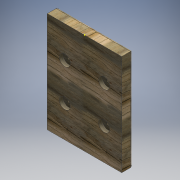
# Autodesk Inventor part: Base
Saved by Autodesk Inventor 2016 (Build 200138000, 138)
## iProperties
Created: 2016-09-10
Part Number: Base
Material: Generic
Document SubType Name: Modeling
Designer: Muhammad
Density: 1 g/cm^3
Appearance: Driftwood
Author: Muhammad
Autodesk Inventor part; units mm, degrees
ref_plane "YZ Plane" through (0, 0, 0) normal (1, 0, 0) x (0, 1, 0)
ref_plane "XZ Plane" through (0, 0, 0) normal (0, 1, 0) x (-1, 0, 0)
ref_plane "XY Plane" through (0, 0, 0) normal (0, 0, 1) x (1, 0, 0)
sketch "Sketch1" plane through (0, 0, 0) normal (0, 1, 0) x (-1, 0, 0)
  line L0 (85, 115) -> (-85, 115)
  line L1 (-85, 115) -> (-85, -115)
  line L2 (-85, -115) -> (85, -115)
  line L3 (85, -115) -> (85, 115)
  line L4 (85, 115) -> (-85, -115) construction
  line L5 (-85, 115) -> (85, -115) construction
  line L6 (-85, 115) -> (-85, 42.5) construction
  line L7 (-85, 42.5) -> (-85, -42.5) construction
  line L8 (-85, 42.5) -> (-45, 42.5) construction
  line L9 (-45, 42.5) -> (45, 42.5) construction
  line L10 (45, 42.5) -> (45, -42.5) construction
  line L11 (-85, -42.5) -> (-45, -42.5) construction
  line L12 (-45, -42.5) -> (45, -42.5) construction
  circle A0 centre (-45, 42.5) radius 3.5
  circle A1 centre (45, 42.5) radius 3.5
  circle A2 centre (45, -42.5) radius 3.5
  line L13 (-45, 42.5) -> (-45, -42.5) construction
  circle A3 centre (-45, -42.5) radius 3.5
  point P0 (0, 0)
  dimension "d3" = 85
  dimension "d7" = 7
  dimension "d8" = 7
  constraints: 28 end point, 4 centre point, 4 coincident, 4 perpendicular, 3 horizontal, 3 point on line, 2 midpoint, 2 parallel
  measures "d3" distance of L6.end L7.end
  measures "d7" diameter of A1
  measures "d8" diameter of A2
extrude "Extrusion1" add sketch "Sketch1" along normal blind 25
sketch "Sketch2" plane through (0, 0, 0) normal (0, -1, 0) x (1, 0, 0)
  circle A0 centre (-45, -42.5) radius 3.5 projected
  circle A1 centre (-45, -42.5) radius 12.5
  circle A2 centre (-45, 42.5) radius 3.5 projected
  circle A3 centre (-45, 42.5) radius 12.5
  circle A4 centre (45, 42.5) radius 3.5 projected
  circle A5 centre (45, 42.5) radius 12.5
  circle A6 centre (45, -42.5) radius 3.5 projected
  circle A7 centre (45, -42.5) radius 12.5
  point P0 (0, 0)
  constraints: 4 centre point, 4 coincident
extrude "Extrusion2" cut sketch "Sketch2" against normal blind 9
sketch "Sketch3" plane through (-85, 0, 115) normal (0, 0, 1) x (1, 0, 0)
  point P0 (85, 0)
sketch "Sketch4" plane through (0, 0, 0) normal (0, 0, 1) x (1, 0, 0)
  line L0 (-85, 0) -> (-85, 25) projected
  line L1 (-85, 7.3168) -> (-67.3168, 25)
  line L2 (-85, 25) -> (85, 25) projected
  line L3 (-85, 7.3168) -> (-59.9922, 7.3168) construction
  point P0 (0, 0)
  dimension "d15" = 45
  constraints: 4 end point, 2 point on line, 1 equal length, 1 horizontal
  measures "d15" angle of L3 L1
extrude "Extrusion3" cut sketch "Sketch4" along normal mid plane 80
fillet "Fillet1" radius 5 5 edges at (85, 25, 0) (0, 25, 115) (-85, 25, 77.5) (-85, 25, -77.5) (0, 25, -115)
body "Solid1"
